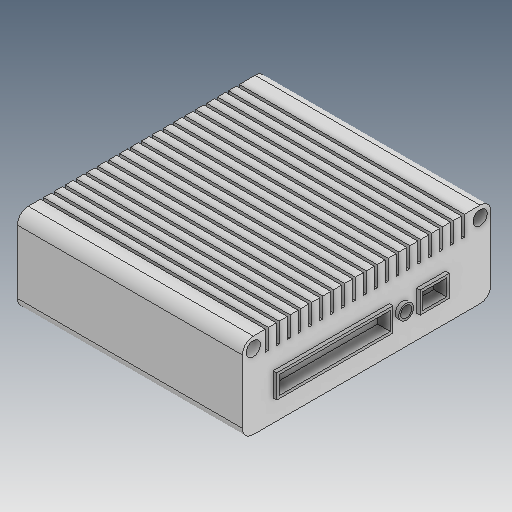
# Autodesk Inventor part: home_lab_router_simplified_model
Saved by Autodesk Inventor 2027 (Build 310192060, 192F)
## iProperties
Created: 2026-07-28
Part Number: home_lab_router_simplified_model
Material: Generic
Document SubType Name: Modeling
Designer: prest
Density: 1 g/cm^3
Appearance: Default
Author: prest
Autodesk Inventor part; units mm, degrees
ref_plane "YZ Plane" through (0, 0, 0) normal (1, 0, 0) x (0, 1, 0)
ref_plane "XZ Plane" through (0, 0, 0) normal (0, 1, 0) x (-1, 0, 0)
ref_plane "XY Plane" through (0, 0, 0) normal (0, 0, 1) x (1, 0, 0)
sketch "Sketch1" plane through (0, 0, 0) normal (0, 1, 0) x (-1, 0, 0)
  line L0 (62, 68.5) -> (-62, 68.5)
  line L1 (-62, 68.5) -> (-62, -68.5)
  line L2 (-62, -68.5) -> (62, -68.5)
  line L3 (62, -68.5) -> (62, 68.5)
  point P0 (0, 0)
  point P1 (0, 68.5)
  point P2 (-62, 0)
  dimension "d0" = 137
  dimension "d1" = 124
  constraints: 8 end point, 2 midpoint, 2 parallel, 1 horizontal, 1 horizontal alignment, 1 perpendicular, 1 vertical alignment
  measures "d0" distance of L2.end L0.start
  measures "d1" distance of L1.end L2.end
extrude "Extrusion1" add sketch "Sketch1" along normal blind 47
fillet "Fillet1" radius 6 4 edges at (0, 47, 68.5) (0, 47, -68.5) (0, 0, -68.5) (0, 0, 68.5)
sketch "Sketch2" plane through (0, 0, 0) normal (0, -1, 0) x (1, 0, 0)
  line L0 (35.75, 0) -> (-35.75, 0) construction
  line L1 (0, 35.75) -> (0, -35.75) construction
  point P0 (0, 0)
  point P1 (0, 0)
  dimension "d5" = 71.5
  dimension "d6" = 71.5
  constraints: 4 end point, 2 midpoint, 2 vertical alignment, 1 coincident, 1 horizontal, 1 horizontal alignment, 1 vertical
  measures "d5" distance of L0.end L0.start
  measures "d6" distance of L1.end L1.start
hole "Hole1" at (-35.75, 0, 0) at (0, 0, 35.75) at (0, 0, -35.75) at (35.75, 0, 0) direction (0, 1, 0) diameter 3.5 depth 4.5 tip angle 118
sketch "Sketch3" plane through (62, 0, 62.5) normal (1, 0, 0) x (0, 0, -1)
  line L0 (11, 25) -> (75, 25)
  line L1 (75, 25) -> (75, 12)
  line L2 (75, 12) -> (11, 12)
  line L3 (11, 12) -> (11, 25)
  line L4 (0, 0) -> (125, 0) projected
  line L5 (-6, 6) -> (-6, 41) projected
  line L6 (131, 6) -> (131, 41) projected
  circle A0 centre (82.2736, 18.5) radius 4.0537
  line L7 (90, 25) -> (106, 25)
  line L8 (106, 25) -> (106, 13)
  line L9 (106, 13) -> (90, 13)
  line L10 (90, 13) -> (90, 25)
  line L11 (104.5, 23.5) -> (91.5, 23.5)
  line L12 (91.5, 23.5) -> (91.5, 14.5)
  line L13 (91.5, 14.5) -> (104.5, 14.5)
  line L14 (104.5, 14.5) -> (104.5, 23.5)
  line L15 (73.5, 23.5) -> (12.5, 23.5)
  line L16 (12.5, 23.5) -> (12.5, 13.5)
  line L17 (12.5, 13.5) -> (73.5, 13.5)
  line L18 (73.5, 13.5) -> (73.5, 23.5)
  circle A1 centre (82.2736, 18.5) radius 3.0537
  point P0 (62.5, 0)
  point P1 (98, 25)
  point P2 (43, 25)
  point P3 (90, 19)
  dimension "d14" = 12
  dimension "d15" = 17
  dimension "d16" = 64
  dimension "d17" = 13
  dimension "d19" = 12
  dimension "d20" = 16
  dimension "d21" = 25
  dimension "d25" = 1.5
  dimension "d26" = 1.5
  dimension "d27" = 1
  constraints: 32 end point, 8 parallel, 4 perpendicular, 3 midpoint, 2 centre point, 2 horizontal, 1 horizontal alignment, 6 other
  measures "d14" distance between parallel lines of L4 L2
  measures "d15" distance between parallel lines of L3 L5
  measures "d16" distance of L1.end L2.end
  measures "d17" distance of L2.end L0.start
  measures "d19" distance of L7.end L8.end
  measures "d20" distance of L8.end L9.end
  measures "d21" distance between parallel lines of L6 L8
  measures "d25" distance between parallel lines of L7 L11
  measures "d26" distance between parallel lines of L0 L15
  measures "d27" radial gap between concentric circles of A0 A1
extrude "Extrusion2" add sketch "Sketch3" along normal blind 2
sketch "Sketch4" plane through (62, 13.5, 50) normal (1, 0, 0) x (0, 0, -1)
  line L0 (61, 10) -> (0, 10) projected
  line L1 (61, 0) -> (0, 0) projected
  line L2 (0, 10) -> (61, 10)
  line L3 (61, 10) -> (61, 0)
  line L4 (61, 0) -> (0, 0)
  line L5 (0, 0) -> (0, 10)
  circle A0 centre (69.7736, 5) radius 3.0537 projected
  circle A1 centre (69.7736, 5) radius 3.0537
  line L6 (92, 1) -> (79, 1) projected
  line L7 (79, 1) -> (92, 1)
  line L8 (92, 1) -> (92, 10)
  line L9 (92, 10) -> (79, 10)
  line L10 (79, 10) -> (79, 1)
  point P0 (50, -13.5)
  constraints: 16 end point, 4 parallel, 2 horizontal, 2 perpendicular, 1 centre point, 1 coincident
extrude "Extrusion3" cut sketch "Sketch4" against normal blind 5
sketch "Sketch5" plane through (62, 0, 62.5) normal (1, 0, 0) x (0, 0, -1)
  line L0 (-6, 6) -> (-6, 41) projected
  line L1 (-6, 36) -> (131, 36)
  line L2 (131, 6) -> (131, 41) projected
  line L3 (0, 0) -> (125, 0) projected
  arc A0 (0, 47) -> (-6, 41) centre (0, 41) ccw projected
  circle A1 centre (0, 41) radius 3.8793
  line L4 (125, 47) -> (0, 47) projected
  line L5 (6.6956, 47) -> (6.6956, 36)
  line L6 (8.2912, 47) -> (8.2912, 36)
  line L7 (0, 36) -> (137, 36)
  line L8 (12.6956, 47) -> (12.6956, 36)
  line L9 (14.2912, 47) -> (14.2912, 36)
  line L10 (6, 36) -> (143, 36)
  line L11 (18.6956, 47) -> (18.6956, 36)
  line L12 (20.2912, 47) -> (20.2912, 36)
  line L13 (12, 36) -> (149, 36)
  line L14 (24.6956, 47) -> (24.6956, 36)
  line L15 (26.2912, 47) -> (26.2912, 36)
  line L16 (18, 36) -> (155, 36)
  line L17 (30.6956, 47) -> (30.6956, 36)
  line L18 (32.2912, 47) -> (32.2912, 36)
  line L19 (24, 36) -> (161, 36)
  line L20 (36.6956, 47) -> (36.6956, 36)
  line L21 (38.2912, 47) -> (38.2912, 36)
  line L22 (30, 36) -> (167, 36)
  line L23 (42.6956, 47) -> (42.6956, 36)
  line L24 (44.2912, 47) -> (44.2912, 36)
  line L25 (36, 36) -> (173, 36)
  line L26 (48.6956, 47) -> (48.6956, 36)
  line L27 (50.2912, 47) -> (50.2912, 36)
  line L28 (42, 36) -> (179, 36)
  line L29 (54.6956, 47) -> (54.6956, 36)
  line L30 (56.2912, 47) -> (56.2912, 36)
  line L31 (48, 36) -> (185, 36)
  line L32 (60.6956, 47) -> (60.6956, 36)
  line L33 (62.2912, 47) -> (62.2912, 36)
  line L34 (54, 36) -> (191, 36)
  line L35 (66.6956, 47) -> (66.6956, 36)
  line L36 (68.2912, 47) -> (68.2912, 36)
  line L37 (60, 36) -> (197, 36)
  line L38 (72.6956, 47) -> (72.6956, 36)
  line L39 (74.2912, 47) -> (74.2912, 36)
  line L40 (66, 36) -> (203, 36)
  line L41 (78.6956, 47) -> (78.6956, 36)
  line L42 (80.2912, 47) -> (80.2912, 36)
  line L43 (72, 36) -> (209, 36)
  line L44 (84.6956, 47) -> (84.6956, 36)
  line L45 (86.2912, 47) -> (86.2912, 36)
  line L46 (78, 36) -> (215, 36)
  line L47 (90.6956, 47) -> (90.6956, 36)
  line L48 (92.2912, 47) -> (92.2912, 36)
  line L49 (84, 36) -> (221, 36)
  line L50 (96.6956, 47) -> (96.6956, 36)
  line L51 (98.2912, 47) -> (98.2912, 36)
  line L52 (90, 36) -> (227, 36)
  line L53 (102.6956, 47) -> (102.6956, 36)
  line L54 (104.2912, 47) -> (104.2912, 36)
  line L55 (96, 36) -> (233, 36)
  line L56 (108.6956, 47) -> (108.6956, 36)
  line L57 (110.2912, 47) -> (110.2912, 36)
  line L58 (102, 36) -> (239, 36)
  line L59 (114.6956, 47) -> (114.6956, 36)
  line L60 (116.2912, 47) -> (116.2912, 36)
  arc A2 (131, 41) -> (125, 47) centre (125, 41) ccw projected
  circle A3 centre (125, 41) radius 3.8793
  point P0 (62.5, 0)
  point P1 (14.2912, 36)
  point P2 (14.2912, 47)
  point P3 (12.6956, 47)
  point P4 (12.6956, 36)
  dimension "d32" = 36
  dimension "d35" = 6
  constraints: 112 end point, 108 horizontal alignment, 38 point on line, 36 parallel, 17 collinear, 2 centre point, 2 coincident, 2 vertical, 1 equal radius, 1 horizontal, 8 other
  measures "d35" distance of point (-6, 36) L7.start
extrude "Extrusion4" cut sketch "Sketch5" against normal through all contours L4 L6 L1 L5 | L4 L9 L1 L8 | L4 L12 L1 L11 | L4 L15 L1 L14 | L4 L18 L1 L17 | L4 L21 L1 L20 | L4 L24 L1 L23 | L4 L27 L1 L26 | L4 L30 L1 L29 | L4 L33 L1 L32 | L4 L36 L1 L35 | L4 L39 L1 L38 | L4 L42 L1 L41 | L4 L45 L1 L44 | L4 L48 L1 L47 | L4 L51 L1 L50 | L4 L54 L1 L53 | L4 L57 L1 L56 | L4 L60 L1 L59 | A1 | A3
body "Solid1"
